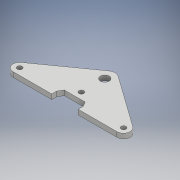
# Autodesk Inventor part: Corpo_Suporte_3_Cabos_Modelo3
Saved by Autodesk Inventor 2018 (Build 220112000, 112)
## iProperties
Created: 2021-08-02
Part Number: Corpo_Suporte_3_Cabos_Modelo3
Material: Generic
Document SubType Name: Modeling
Designer: L08619
Density: 1 g/cm^3
Appearance: Default
Author: L08619
Autodesk Inventor part; units mm, degrees
ref_plane "YZ Plane" through (0, 0, 0) normal (1, 0, 0) x (0, 1, 0)
ref_plane "XZ Plane" through (0, 0, 0) normal (0, 1, 0) x (-1, 0, 0)
ref_plane "XY Plane" through (0, 0, 0) normal (0, 0, 1) x (1, 0, 0)
sketch "Sketch1" plane through (0, 0, 0) normal (0, 0, 1) x (1, 0, 0)
  circle A0 centre (0, 0) radius 20
  circle A1 centre (-235, -150) radius 11
  line L0 (-20.1258, 40) -> (-10.1258, 46.2314) construction
  spline S0 degree 2 poles (-20.1258, 40) (-10.1258, 46.2314) (0, 46.2314) knots 1 1 1 1.5 1.5 1.5
  line L1 (0, 87.1559) -> (0, -290.9336) construction
  line L2 (-10.1258, 46.2314) -> (0, 46.2314) construction
  circle A2 centre (235, -150) radius 11
  line L3 (20.1258, 40) -> (10.1258, 46.2314) construction
  spline S1 degree 2 poles (20.1258, 40) (10.1258, 46.2314) (0, 46.2314) knots 1 1 1 1.5 1.5 1.5
  line L4 (10.1258, 46.2314) -> (0, 46.2314) construction
  circle A3 centre (0, -106) radius 11
  line L5 (-60, -180) -> (-60, -158)
  line L6 (-47.2983, -136) -> (47.2983, -136)
  line L7 (60, -158) -> (60, -180)
  line L8 (-60, -158) -> (-47.2983, -136)
  line L9 (-60, -158) -> (-34.5966, -158) construction
  line L10 (60, -158) -> (47.2983, -136)
  line L11 (60, -158) -> (85.4034, -158) construction
  line L12 (-60, -180) -> (-235, -180)
  arc A4 (-252.4129, -125.5707) -> (-235, -180) centre (-235, -150) ccw
  arc A5 (-252.4129, -125.5707) -> (-252.4129, -125.5707) centre (-235, -150) ccw
  line L13 (60, -180) -> (235, -180)
  arc A6 (235, -180) -> (252.4129, -125.5707) centre (235, -150) ccw
  arc A7 (252.4129, -125.5707) -> (252.4129, -125.5707) centre (235, -150) ccw
  line L14 (-20.1258, 40) -> (-252.4129, -125.5707)
  line L15 (20.1258, 40) -> (252.4129, -125.5707)
  dimension "d0" = 40
  dimension "d3" = 22
  dimension "d9" = 40
  dimension "d16" = 22
  dimension "d18" = 235
  dimension "d19" = 30
  dimension "d21" = 120
  dimension "d23" = 60
  dimension "d24" = 235
  dimension "d25" = 60
  dimension "d26" = 120
  constraints: 24 end point, 10 point on circle, 9 symmetric about line, 8 centre point, 3 horizontal, 3 tangent, 2 concentric, 2 equal length, 2 perpendicular, 2 point on line, 1 coincident, 1 horizontal alignment, 1 vertical, 9 other
  measures "d0" diameter of A0
  measures "d3" diameter of A1
  measures "d9" vertical distance of L0.start point (0, 0)
  measures "d16" diameter of A3
  measures "d18" horizontal distance of A1.centre point (0, 0)
  measures "d19" distance from line of A3.centre L6
  measures "d21" distance between parallel lines of L5 L7
  measures "d23" distance from line of A3.centre L7
  measures "d24" horizontal distance of A2.centre point (0, 0)
  measures "d25" angle of L9 L8
  measures "d26" angle of L11 L10
extrude "Extrusion2" add sketch "Sketch1" along normal mid plane 22.22
body "Solid2"
